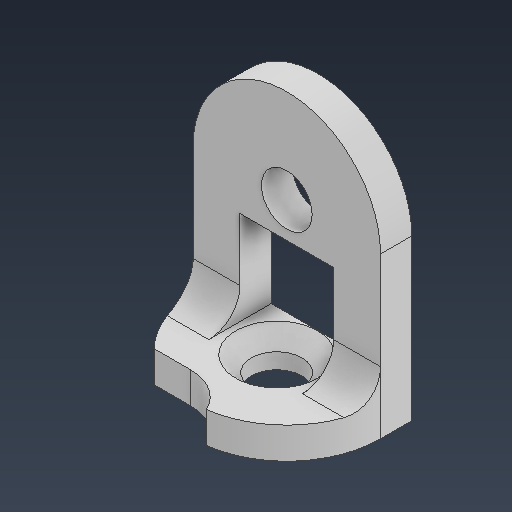
# Autodesk Inventor part: уголок смешной
Saved by Autodesk Inventor 2026 (Build 300175000, 175)
## iProperties
Created: 2026-01-11
Part Number: уголок смешной
Material: Типовые
Document SubType Name: Modeling
Designer: GameHD
Density: 1 g/cm^3
Appearance: По умолчанию
Author: GameHD
Autodesk Inventor part; units mm, degrees
(part 1 of 2)
ref_plane "YZ Plane" through (0, 0, 0) normal (1, 0, 0) x (0, 1, 0)
ref_plane "XZ Plane" through (0, 0, 0) normal (0, 1, 0) x (-1, 0, 0)
ref_plane "XY Plane" through (0, 0, 0) normal (0, 0, 1) x (1, 0, 0)
sketch "Эскиз1" plane through (0, 0, 0) normal (0, 0, 1) x (1, 0, 0)
  circle A0 centre (0, 0) radius 1.625
  line L0 (0, 0) -> (0, -10.25)
  line L1 (-6, 6) -> (6, 6)
  line L2 (6, 6) -> (6, -10.25)
  line L3 (6, -10.25) -> (-6, -10.25)
  line L4 (-6, -10.25) -> (-6, 6)
  line L5 (0, -10.25) -> (-3, -10.25)
  line L6 (-3, -10.25) -> (-3, -4.25)
  line L7 (-3, -4.25) -> (0, -4.25)
  line L8 (0, -4.25) -> (0, -10.25)
  line L9 (3, -10.25) -> (3, -4.25)
  line L10 (3, -4.25) -> (0, -4.25)
  dimension "d0" = 3.25
  dimension "d1" = 10.25
  dimension "d2" = 6
  dimension "d3" = 6
  dimension "d4" = 6
  dimension "d5" = 10.25
  dimension "d6" = 3
  dimension "d7" = 6
  constraints: 22 end point, 4 parallel, 2 horizontal, 2 perpendicular, 2 symmetric about line, 1 centre point, 1 coincident, 1 vertical
  measures "d0" diameter of A0
  measures "d1" distance of L0.start L0.end
  measures "d2" distance from line of L2 L0.start
  measures "d3" distance from line of L4 L0.start
  measures "d4" distance from line of L0.start L1
  measures "d5" distance from line of L0.start L3
  measures "d6" distance of L6.end L7.end
  measures "d7" distance of L5.end L6.end
extrude "Выдавливание1" add sketch "Эскиз1" along normal blind 2 contours L7 L6 L3 L4 L1 L2 L9 L10
sketch "Эскиз2" plane through (0, 0, 2) normal (0, 0, 1) x (1, 0, 0)
  line L0 (3, -4.25) -> (3, -10.25) projected
  line L1 (3, -10.25) -> (6, -10.25) projected
  line L2 (6, -10.25) -> (6, 6) projected
  line L3 (6, 6) -> (-6, 6) projected
  line L4 (-6, 6) -> (-6, -10.25) projected
  line L5 (-6, -10.25) -> (-3, -10.25) projected
  line L6 (-3, -10.25) -> (-3, -4.25) projected
  line L7 (-3, -4.25) -> (3, -4.25) projected
  circle A0 centre (0, 0) radius 1.625 projected
  line L8 (-6, -10.25) -> (6, -10.25)
  line L9 (6, -10.25) -> (6, -8.25)
  line L10 (6, -8.25) -> (-6, -8.25)
  line L11 (-6, -8.25) -> (-6, -10.25)
  dimension "d10" = 12
  dimension "d11" = 2
  constraints: 8 end point, 2 parallel, 1 horizontal, 1 perpendicular
  measures "d10" distance of L10.end L9.end
  measures "d11" distance of L9.end L8.end
extrude "Выдавливание2" add sketch "Эскиз2" along normal blind 6 and the other way blind 2 contours L10 L2 L1 L0 | L0 L8 L6 L10 | L6 L5 L4 L10
sketch "Эскиз3" plane through (-6, -8.25, 2) normal (0, 1, 0) x (1, 0, 0)
  line L0 (0, 0) -> (3, 0) projected
  line L1 (0, -6) -> (0, 0) projected
  line L2 (12, -6) -> (0, -6) projected
  line L3 (12, 0) -> (12, -6) projected
  line L4 (9, 0) -> (12, 0) projected
  line L5 (9, 2) -> (9, 0) projected
  line L6 (3, 2) -> (9, 2) projected
  line L7 (3, 0) -> (3, 2) projected
  circle A0 centre (6, -0.65) radius 1.625
  line L8 (12, 2) -> (0, 2) projected
  point P0 (6, 2)
  point P1 (6, 2)
  dimension "d16" = 3.25
  dimension "d17" = 2.65
  dimension "d20" = 0
  constraints: 1 centre point, 1 midpoint
  measures "d16" diameter of A0
  measures "d17" distance from line of L6 A0.centre
  measures "d20" horizontal distance of point (6, 2) A0.centre
extrude "Выдавливание3" cut sketch "Эскиз3" against normal blind 3.25 contours A0
chamfer "Фаска1" distance 1 angle 45 1 edges at (-1.625, -8.25, 2.65)
fillet "Сопряжение1" radius 6 2 edges at (-6, -9.25, 8) (6, -9.25, 8)
sketch "Эскиз4" plane through (-3, -8.25, 0) normal (0, 1, 0) x (1, 0, 0)
  arc A0 (-244.3999, -16) -> (-248.3999, -20) centre (-244.3999, -20) ccw construction
  line L0 (-244.3999, -16) -> (-177.3999, -16) construction
  arc A1 (-173.3999, -20) -> (-177.3999, -16) centre (-177.3999, -20) ccw construction
  line L1 (-173.3999, -20) -> (-173.3999, -62) construction
  arc A2 (-177.3999, -66) -> (-173.3999, -62) centre (-177.3999, -62) ccw construction
  line L2 (-177.3999, -66) -> (-244.3999, -66) construction
  arc A3 (-248.3999, -62) -> (-244.3999, -66) centre (-244.3999, -62) ccw construction
  line L3 (-248.3999, -62) -> (-248.3999, -20) construction
  line L4 (-244.3999, -336.5) -> (-177.3999, -336.5) construction
  arc A4 (-173.3999, -340.5) -> (-177.3999, -336.5) centre (-177.3999, -340.5) ccw construction
  line L5 (-173.3999, -340.5) -> (-173.3999, -382.5) construction
  arc A5 (-177.3999, -386.5) -> (-173.3999, -382.5) centre (-177.3999, -382.5) ccw construction
  line L6 (-177.3999, -386.5) -> (-244.3999, -386.5) construction
  arc A6 (-248.3999, -382.5) -> (-244.3999, -386.5) centre (-244.3999, -382.5) ccw construction
  line L7 (-248.3999, -382.5) -> (-248.3999, -340.5) construction
  arc A7 (-244.3999, -336.5) -> (-248.3999, -340.5) centre (-244.3999, -340.5) ccw construction
  arc A8 (-136.2796, -72.3282) -> (-139.52, -72.3282) centre (-137.8998, -72.2032) ccw construction
  arc A9 (-139.52, -72.3282) -> (-136.2796, -72.3282) centre (-137.8998, -72.4532) ccw construction
  arc A10 (-365.52, -89.5782) -> (-362.2796, -89.5782) centre (-363.8998, -89.7032) ccw construction
  arc A11 (-362.2796, -89.5782) -> (-365.52, -89.5782) centre (-363.8998, -89.4532) ccw construction
  arc A12 (-225.52, -330.1718) -> (-222.2796, -330.1718) centre (-223.8998, -330.2968) ccw construction
  arc A13 (-222.2796, -330.1718) -> (-225.52, -330.1718) centre (-223.8998, -330.0468) ccw construction
  arc A14 (0.4798, -330.1718) -> (3.7202, -330.1718) centre (2.1, -330.2968) ccw construction
  arc A15 (3.7202, -330.1718) -> (0.4798, -330.1718) centre (2.1, -330.0468) ccw construction
  arc A16 (-136.2796, -312.9218) -> (-139.52, -312.9218) centre (-137.8998, -312.7968) ccw construction
  arc A17 (-139.52, -312.9218) -> (-136.2796, -312.9218) centre (-137.8998, -313.0468) ccw construction
  arc A18 (-362.2796, -312.9218) -> (-365.52, -312.9218) centre (-363.8998, -312.7968) ccw construction
  arc A19 (-365.52, -312.9218) -> (-362.2796, -312.9218) centre (-363.8998, -313.0468) ccw construction
  arc A20 (-225.52, -89.5782) -> (-222.2796, -89.5782) centre (-223.8998, -89.7032) ccw construction
  arc A21 (-222.2796, -89.5782) -> (-225.52, -89.5782) centre (-223.8998, -89.4532) ccw construction
  arc A22 (0.4798, -89.5782) -> (3.7202, -89.5782) centre (2.1, -89.7032) ccw construction
  arc A23 (3.7202, -89.5782) -> (0.4798, -89.5782) centre (2.1, -89.4532) ccw construction
  arc A24 (-139.52, -89.5782) -> (-136.2796, -89.5782) centre (-137.8998, -89.7032) ccw construction
  arc A25 (-136.2796, -89.5782) -> (-139.52, -89.5782) centre (-137.8998, -89.4532) ccw construction
  arc A26 (-362.2796, -72.3282) -> (-365.52, -72.3282) centre (-363.8998, -72.2032) ccw construction
  arc A27 (-365.52, -72.3282) -> (-362.2796, -72.3282) centre (-363.8998, -72.4532) ccw construction
  arc A28 (-222.2796, -312.9218) -> (-225.52, -312.9218) centre (-223.8998, -312.7968) ccw construction
  arc A29 (-225.52, -312.9218) -> (-222.2796, -312.9218) centre (-223.8998, -313.0468) ccw construction
  arc A30 (3.7202, -312.9218) -> (0.4798, -312.9218) centre (2.1, -312.7968) ccw construction
  arc A31 (0.4798, -312.9218) -> (3.7202, -312.9218) centre (2.1, -313.0468) ccw construction
  arc A32 (-139.52, -330.1718) -> (-136.2796, -330.1718) centre (-137.8998, -330.2968) ccw construction
  arc A33 (-136.2796, -330.1718) -> (-139.52, -330.1718) centre (-137.8998, -330.0468) ccw construction
  arc A34 (-365.52, -330.1718) -> (-362.2796, -330.1718) centre (-363.8998, -330.2968) ccw construction
  arc A35 (-362.2796, -330.1718) -> (-365.52, -330.1718) centre (-363.8998, -330.0468) ccw construction
  arc A36 (-222.2796, -72.3282) -> (-225.52, -72.3282) centre (-223.8998, -72.2032) ccw construction
  arc A37 (-225.52, -72.3282) -> (-222.2796, -72.3282) centre (-223.8998, -72.4532) ccw construction
  arc A38 (3.7202, -72.3282) -> (0.4798, -72.3282) centre (2.1, -72.2032) ccw construction
  arc A39 (0.4798, -72.3282) -> (3.7202, -72.3282) centre (2.1, -72.4532) ccw construction
  circle A40 centre (-364.7998, -2.65) radius 1.625 construction
  circle A41 centre (-364.8998, -399.85) radius 1.625 construction
  circle A42 centre (3.0002, -2.65) radius 1.625 construction
  circle A43 centre (3.0002, -399.85) radius 1.625 construction
  circle A44 centre (-180.9846, -7.75) radius 1.625 construction
  circle A45 centre (-180.9846, -394.75) radius 1.625 construction
  circle A46 centre (-223.8998, -7.75) radius 1.625 construction
  circle A47 centre (-223.8998, -394.75) radius 1.625 construction
  circle A48 centre (-124.9057, -203.075) radius 1.85 construction
  arc A49 (-189.2088, -201.25) -> (-188.6026, -201.25) centre (-188.9057, -203.075) ccw construction
  line L8 (-189.2088, -201.25) -> (-188.6026, -201.25) construction
  circle A50 centre (-124.9057, -261.875) radius 2 construction
  circle A51 centre (-308.8939, -169) radius 2.1 construction
  circle A52 centre (-52.9057, -233.5) radius 2.1 construction
  circle A53 centre (-113.9057, -233.5) radius 2.1 construction
  circle A54 centre (-308.8939, -233.5) radius 2.1 construction
  circle A55 centre (-247.8939, -169) radius 2.1 construction
  circle A56 centre (-52.9057, -169) radius 2.1 construction
  circle A57 centre (-113.9057, -169) radius 2.1 construction
  circle A58 centre (-247.8939, -233.5) radius 2.1 construction
  line L9 (-39.8998, -221.25) -> (-3.8998, -221.25) construction
  arc A59 (-0.8998, -224.25) -> (-3.8998, -221.25) centre (-3.8998, -224.25) ccw construction
  line L10 (-0.8998, -224.25) -> (-0.8998, -290.25) construction
  arc A60 (-3.8998, -293.25) -> (-0.8998, -290.25) centre (-3.8998, -290.25) ccw construction
  line L11 (-3.8998, -293.25) -> (-39.8998, -293.25) construction
  arc A61 (-42.8998, -290.25) -> (-39.8998, -293.25) centre (-39.8998, -290.25) ccw construction
  line L12 (-42.8998, -290.25) -> (-42.8998, -224.25) construction
  arc A62 (-39.8998, -221.25) -> (-42.8998, -224.25) centre (-39.8998, -224.25) ccw construction
  circle A63 centre (-160.9, -67.1372) radius 2.1 construction
  circle A64 centre (-52.2429, -99.25) radius 2.1 construction
  circle A65 centre (-160.9, -335.3628) radius 2.1 construction
  circle A66 centre (-52.2429, -212.2592) radius 2.1 construction
  circle A67 centre (-55.8998, -251) radius 2.1 construction
  circle A68 centre (-55.8998, -283.25) radius 2.1 construction
  arc A69 (-25.0518, -344.25) -> (-23.0518, -346.25) centre (-23.0518, -344.25) ccw construction
  line L13 (-23.0518, -346.25) -> (1.1002, -346.25) construction
  arc A70 (4.1002, -349.25) -> (1.1002, -346.25) centre (1.1002, -349.25) ccw construction
  line L14 (4.1002, -349.25) -> (4.1002, -393.25) construction
  arc A71 (1.1002, -396.25) -> (4.1002, -393.25) centre (1.1002, -393.25) ccw construction
  line L15 (1.1002, -396.25) -> (-155.8998, -396.25) construction
  arc A72 (-158.8998, -393.25) -> (-155.8998, -396.25) centre (-155.8998, -393.25) ccw construction
  line L16 (-158.8998, -393.25) -> (-158.8998, -349.25) construction
  arc A73 (-155.8998, -346.25) -> (-158.8998, -349.25) centre (-155.8998, -349.25) ccw construction
  line L17 (-155.8998, -346.25) -> (-107.0518, -346.25) construction
  arc A74 (-107.0518, -346.25) -> (-105.0518, -344.25) centre (-107.0518, -344.25) ccw construction
  line L18 (-105.0518, -344.25) -> (-105.0518, -332.25) construction
  arc A75 (-103.0518, -330.25) -> (-105.0518, -332.25) centre (-103.0518, -332.25) ccw construction
  line L19 (-103.0518, -330.25) -> (-27.0518, -330.25) construction
  arc A76 (-25.0518, -332.25) -> (-27.0518, -330.25) centre (-27.0518, -332.25) ccw construction
  line L20 (-25.0518, -332.25) -> (-25.0518, -344.25) construction
  arc A77 (-338.7478, -346.25) -> (-336.7478, -344.25) centre (-338.7478, -344.25) ccw construction
  line L21 (-336.7478, -344.25) -> (-336.7478, -332.25) construction
  arc A78 (-334.7478, -330.25) -> (-336.7478, -332.25) centre (-334.7478, -332.25) ccw construction
  line L22 (-334.7478, -330.25) -> (-258.7478, -330.25) construction
  arc A79 (-256.7478, -332.25) -> (-258.7478, -330.25) centre (-258.7478, -332.25) ccw construction
  line L23 (-256.7478, -332.25) -> (-256.7478, -394.25) construction
  arc A80 (-258.7478, -396.25) -> (-256.7478, -394.25) centre (-258.7478, -394.25) ccw construction
  line L24 (-258.7478, -396.25) -> (-362.8998, -396.25) construction
  arc A81 (-365.8998, -393.25) -> (-362.8998, -396.25) centre (-362.8998, -393.25) ccw construction
  line L25 (-365.8998, -393.25) -> (-365.8998, -349.25) construction
  arc A82 (-362.8998, -346.25) -> (-365.8998, -349.25) centre (-362.8998, -349.25) ccw construction
  line L26 (-362.8998, -346.25) -> (-338.7478, -346.25) construction
  arc A83 (-336.7478, -58.25) -> (-338.7478, -56.25) centre (-338.7478, -58.25) ccw construction
  line L27 (-338.7478, -56.25) -> (-362.8998, -56.25) construction
  arc A84 (-365.8998, -53.25) -> (-362.8998, -56.25) centre (-362.8998, -53.25) ccw construction
  line L28 (-365.8998, -53.25) -> (-365.8998, -9.25) construction
  arc A85 (-362.8998, -6.25) -> (-365.8998, -9.25) centre (-362.8998, -9.25) ccw construction
  line L29 (-362.8998, -6.25) -> (-258.7478, -6.25) construction
  arc A86 (-256.7478, -8.25) -> (-258.7478, -6.25) centre (-258.7478, -8.25) ccw construction
  line L30 (-256.7478, -8.25) -> (-256.7478, -70.25) construction
  arc A87 (-258.7478, -72.25) -> (-256.7478, -70.25) centre (-258.7478, -70.25) ccw construction
  line L31 (-258.7478, -72.25) -> (-334.7478, -72.25) construction
  arc A88 (-336.7478, -70.25) -> (-334.7478, -72.25) centre (-334.7478, -70.25) ccw construction
  line L32 (-336.7478, -70.25) -> (-336.7478, -58.25) construction
  arc A89 (-23.0518, -56.25) -> (-25.0518, -58.25) centre (-23.0518, -58.25) ccw construction
  line L33 (-25.0518, -58.25) -> (-25.0518, -70.25) construction
  arc A90 (-27.0518, -72.25) -> (-25.0518, -70.25) centre (-27.0518, -70.25) ccw construction
  line L34 (-27.0518, -72.25) -> (-103.0518, -72.25) construction
  arc A91 (-105.0518, -70.25) -> (-103.0518, -72.25) centre (-103.0518, -70.25) ccw construction
  line L35 (-105.0518, -70.25) -> (-105.0518, -58.25) construction
  arc A92 (-105.0518, -58.25) -> (-107.0518, -56.25) centre (-107.0518, -58.25) ccw construction
  line L36 (-107.0518, -56.25) -> (-155.8998, -56.25) construction
  arc A93 (-158.8998, -53.25) -> (-155.8998, -56.25) centre (-155.8998, -53.25) ccw construction
  line L37 (-158.8998, -53.25) -> (-158.8998, -9.25) construction
  arc A94 (-155.8998, -6.25) -> (-158.8998, -9.25) centre (-155.8998, -9.25) ccw construction
  line L38 (-155.8998, -6.25) -> (1.1002, -6.25) construction
  arc A95 (4.1002, -9.25) -> (1.1002, -6.25) centre (1.1002, -9.25) ccw construction
  line L39 (4.1002, -9.25) -> (4.1002, -53.25) construction
  arc A96 (1.1002, -56.25) -> (4.1002, -53.25) centre (1.1002, -53.25) ccw construction
  line L40 (1.1002, -56.25) -> (-23.0518, -56.25) construction
  line L41 (-167.0538, -195.3437) -> (-132.3026, -179.5551) construction
  arc A97 (-128.7277, -184.1712) -> (-132.3026, -179.5551) centre (-131.0617, -182.2864) ccw construction
  line L42 (-128.7277, -184.1712) -> (-141.4776, -199.9598) construction
  arc A98 (-143.8116, -201.075) -> (-141.4776, -199.9598) centre (-143.8116, -198.075) ccw construction
  line L43 (-143.8116, -201.075) -> (-165.8128, -201.075) construction
  arc A99 (-167.0538, -195.3437) -> (-165.8128, -201.075) centre (-165.8128, -198.075) ccw construction
  line L44 (-155.8716, -230.7092) -> (-156.8392, -229.8202) construction
  arc A100 (-157.1435, -225.7262) -> (-156.8392, -229.8202) centre (-154.8095, -227.611) ccw construction
  line L45 (-157.1435, -225.7262) -> (-141.3675, -206.1902) construction
  arc A101 (-139.0335, -205.075) -> (-141.3675, -206.1902) centre (-139.0335, -208.075) ccw construction
  line L46 (-139.0335, -205.075) -> (-136.3621, -205.075) construction
  arc A102 (-133.6126, -206.875) -> (-136.3621, -205.075) centre (-136.3621, -208.075) ccw construction
  arc A103 (-133.6126, -206.875) -> (-128.7057, -211.7819) centre (-124.9057, -203.075) ccw construction
  arc A104 (-126.9057, -214.5314) -> (-128.7057, -211.7819) centre (-129.9057, -214.5314) ccw construction
  line L47 (-126.9057, -214.5314) -> (-126.9057, -228.5) construction
  arc A105 (-129.9057, -231.5) -> (-126.9057, -228.5) centre (-129.9057, -228.5) ccw construction
  line L48 (-129.9057, -231.5) -> (-153.8419, -231.5) construction
  arc A106 (-155.8716, -230.7092) -> (-153.8419, -231.5) centre (-153.8419, -228.5) ccw construction
  line L49 (-181.876, -212.2495) -> (-166.5929, -226.2908) construction
  arc A107 (-168.6226, -231.5) -> (-166.5929, -226.2908) centre (-168.6226, -228.5) ccw construction
  line L50 (-168.6226, -231.5) -> (-183.9057, -231.5) construction
  arc A108 (-186.9057, -228.5) -> (-183.9057, -231.5) centre (-183.9057, -228.5) ccw construction
  line L51 (-186.9057, -228.5) -> (-186.9057, -214.4586) construction
  arc A109 (-181.876, -212.2495) -> (-186.9057, -214.4586) centre (-183.9057, -214.4586) ccw construction
  line L52 (-65.9033, -278.0576) -> (-103.7626, -266.3304) construction
  arc A110 (-103.342, -260.5013) -> (-103.7626, -266.3304) centre (-102.875, -263.4648) ccw construction
  line L53 (-103.342, -260.5013) -> (-65.4826, -254.5349) construction
  arc A111 (-62.0156, -257.4983) -> (-65.4826, -254.5349) centre (-65.0156, -257.4983) ccw construction
  line L54 (-62.0156, -257.4983) -> (-62.0156, -275.192) construction
  arc A112 (-65.9033, -278.0576) -> (-62.0156, -275.192) centre (-65.0156, -275.192) ccw construction
  line L55 (-264.0269, -167) -> (-296.2344, -167) construction
  arc A113 (-298.2843, -161.8097) -> (-296.2344, -167) centre (-296.2344, -164) ccw construction
  line L56 (-298.2843, -161.8097) -> (-284.6652, -149.0634) construction
  arc A114 (-280.9187, -148.7796) -> (-284.6652, -149.0634) centre (-282.6152, -151.2537) ccw construction
  line L57 (-280.9187, -148.7796) -> (-262.3303, -161.5258) construction
  arc A115 (-264.0269, -167) -> (-262.3303, -161.5258) centre (-264.0269, -164) ccw construction
  line L58 (-228.6675, -225.8338) -> (-198.1708, -210.1041) construction
  arc A116 (-194.902, -210.4435) -> (-198.1708, -210.1041) centre (-196.7956, -212.7703) ccw construction
  arc A117 (-194.902, -210.4435) -> (-192.7057, -211.7819) centre (-188.9057, -203.075) ccw construction
  arc A118 (-190.9057, -214.5314) -> (-192.7057, -211.7819) centre (-193.9057, -214.5314) ccw construction
  line L59 (-190.9057, -214.5314) -> (-190.9057, -228.5) construction
  arc A119 (-193.9057, -231.5) -> (-190.9057, -228.5) centre (-193.9057, -228.5) ccw construction
  line L60 (-193.9057, -231.5) -> (-227.2924, -231.5) construction
  arc A120 (-228.6675, -225.8338) -> (-227.2924, -231.5) centre (-227.2924, -228.5) ccw construction
  line L61 (-162.65, -104.8841) -> (-179.1418, -116.8109) construction
  arc A121 (-182.6579, -116.8109) -> (-179.1418, -116.8109) centre (-180.8998, -114.3799) ccw construction
  line L62 (-182.6579, -116.8109) -> (-206.6593, -99.4532) construction
  line L63 (-206.6593, -99.4532) -> (-164.408, -99.4532) construction
  arc A122 (-162.65, -104.8841) -> (-164.408, -99.4532) centre (-164.408, -102.4532) ccw construction
  line L64 (-256.2113, -160.8716) -> (-276.8346, -146.7299) construction
  arc A123 (-277.188, -142.0654) -> (-276.8346, -146.7299) centre (-275.138, -144.2558) ccw construction
  line L65 (-277.188, -142.0654) -> (-236.1047, -103.6152) construction
  arc A124 (-231.1826, -106.6719) -> (-236.1047, -103.6152) centre (-234.0548, -105.8056) ccw construction
  line L66 (-231.1826, -106.6719) -> (-246.5003, -157.4541) construction
  arc A125 (-249.0176, -159.5667) -> (-246.5003, -157.4541) centre (-249.3725, -156.5878) ccw construction
  arc A126 (-249.0176, -159.5667) -> (-252.9258, -160.942) centre (-247.8939, -169) ccw construction
  arc A127 (-256.2113, -160.8716) -> (-252.9258, -160.942) centre (-254.5148, -158.3974) ccw construction
  arc A128 (-65.5653, -167) -> (-63.5153, -161.8097) centre (-65.5653, -164) ccw construction
  line L67 (-65.5653, -167) -> (-102.8117, -167) construction
  arc A129 (-105.0593, -162.013) -> (-102.8117, -167) centre (-102.8117, -164) ccw construction
  line L68 (-105.0593, -162.013) -> (-88.1952, -142.9371) construction
  arc A130 (-83.8976, -142.7337) -> (-88.1952, -142.9371) centre (-85.9475, -144.9241) ccw construction
  line L69 (-83.8976, -142.7337) -> (-63.5153, -161.8097) construction
  line L70 (-243.0573, -104.6436) -> (-281.5342, -140.6545) construction
  arc A131 (-285.2808, -140.9383) -> (-281.5342, -140.6545) centre (-283.5842, -138.4641) ccw construction
  line L71 (-285.2808, -140.9383) -> (-307.5905, -125.6402) construction
  arc A132 (-308.8939, -123.166) -> (-307.5905, -125.6402) centre (-305.8939, -123.166) ccw construction
  line L72 (-308.8939, -123.166) -> (-308.8939, -102.4532) construction
  arc A133 (-305.8939, -99.4532) -> (-308.8939, -102.4532) centre (-305.8939, -102.4532) ccw construction
  line L73 (-305.8939, -99.4532) -> (-245.1073, -99.4532) construction
  arc A134 (-243.0573, -104.6436) -> (-245.1073, -99.4532) centre (-245.1073, -102.4532) ccw construction
  line L74 (-187.6741, -122.9814) -> (-203.7515, -134.6084) construction
  arc A135 (-208.3766, -133.0605) -> (-203.7515, -134.6084) centre (-205.5095, -132.1774) ccw construction
  line L75 (-208.3766, -133.0605) -> (-217.5313, -103.3362) construction
  arc A136 (-214.6642, -99.4532) -> (-217.5313, -103.3362) centre (-214.6642, -102.4532) ccw construction
  line L76 (-214.6642, -99.4532) -> (-214.4563, -99.4532) construction
  arc A137 (-212.6983, -100.0223) -> (-214.4563, -99.4532) centre (-214.4563, -102.4532) ccw construction
  line L77 (-212.6983, -100.0223) -> (-187.6741, -118.1195) construction
  arc A138 (-187.6741, -122.9814) -> (-187.6741, -118.1195) centre (-189.4322, -120.5504) ccw construction
  line L78 (-200.0044, -206.5491) -> (-238.6289, -226.4709) construction
  arc A139 (-241.8976, -226.1315) -> (-238.6289, -226.4709) centre (-240.0041, -223.8047) ccw construction
  arc A140 (-241.8976, -226.1315) -> (-244.0939, -224.7931) centre (-247.8939, -233.5) ccw construction
  arc A141 (-245.8939, -222.0436) -> (-244.0939, -224.7931) centre (-242.8939, -222.0436) ccw construction
  line L79 (-245.8939, -222.0436) -> (-245.8939, -180.4564) construction
  arc A142 (-244.0939, -177.7069) -> (-245.8939, -180.4564) centre (-242.8939, -180.4564) ccw construction
  arc A143 (-244.0939, -177.7069) -> (-242.2553, -176.6456) centre (-247.8939, -169) ccw construction
  arc A144 (-238.9741, -176.4623) -> (-242.2553, -176.6456) centre (-240.4747, -179.0601) ccw construction
  line L80 (-238.9741, -176.4623) -> (-199.8263, -199.0763) construction
  arc A145 (-198.3458, -202.0103) -> (-199.8263, -199.0763) centre (-201.3269, -201.674) ccw construction
  arc A146 (-198.3458, -202.0103) -> (-198.3858, -203.689) centre (-188.9057, -203.075) ccw construction
  arc A147 (-200.0044, -206.5491) -> (-198.3858, -203.689) centre (-201.3796, -203.8829) ccw construction
  line L81 (-281.5342, -261.8455) -> (-240.9203, -299.8564) construction
  arc A148 (-242.9703, -305.0468) -> (-240.9203, -299.8564) centre (-242.9703, -302.0468) ccw construction
  line L82 (-242.9703, -305.0468) -> (-305.8939, -305.0468) construction
  arc A149 (-308.8939, -302.0468) -> (-305.8939, -305.0468) centre (-305.8939, -302.0468) ccw construction
  line L83 (-308.8939, -302.0468) -> (-308.8939, -279.334) construction
  arc A150 (-307.5905, -276.8598) -> (-308.8939, -279.334) centre (-305.8939, -279.334) ccw construction
  line L84 (-307.5905, -276.8598) -> (-285.2808, -261.5617) construction
  arc A151 (-281.5342, -261.8455) -> (-285.2808, -261.5617) centre (-283.5842, -264.0359) ccw construction
  line L85 (-249.8939, -181.5636) -> (-249.8939, -220.9364) construction
  arc A152 (-255.0736, -222.9977) -> (-249.8939, -220.9364) centre (-252.8939, -220.9364) ccw construction
  line L86 (-255.0736, -222.9977) -> (-273.6917, -203.3114) construction
  arc A153 (-273.6917, -199.1886) -> (-273.6917, -203.3114) centre (-271.512, -201.25) ccw construction
  line L87 (-273.6917, -199.1886) -> (-255.0736, -179.5023) construction
  arc A154 (-249.8939, -181.5636) -> (-255.0736, -179.5023) centre (-252.8939, -181.5636) ccw construction
  line L88 (-64.5486, -250.3383) -> (-80.3123, -252.8226) construction
  arc A155 (-81.8793, -247.0681) -> (-80.3123, -252.8226) centre (-80.7793, -249.8592) ccw construction
  line L89 (-81.8793, -247.0681) -> (-66.1156, -240.8557) construction
  arc A156 (-62.0156, -243.6467) -> (-66.1156, -240.8557) centre (-65.0156, -243.6467) ccw construction
  line L90 (-62.0156, -243.6467) -> (-62.0156, -247.3749) construction
  arc A157 (-64.5486, -250.3383) -> (-62.0156, -247.3749) centre (-65.0156, -247.3749) ccw construction
  line L91 (-126.9057, -238.5) -> (-126.9057, -250.4914) construction
  arc A158 (-131.9354, -252.7005) -> (-126.9057, -250.4914) centre (-129.9057, -250.4914) ccw construction
  line L92 (-131.9354, -252.7005) -> (-144.9872, -240.7092) construction
  arc A159 (-142.9575, -235.5) -> (-144.9872, -240.7092) centre (-142.9575, -238.5) ccw construction
  line L93 (-142.9575, -235.5) -> (-129.9057, -235.5) construction
  arc A160 (-126.9057, -238.5) -> (-129.9057, -235.5) centre (-129.9057, -238.5) ccw construction
  line L94 (-178.5975, -175.2286) -> (-185.296, -190.1505) construction
  arc A161 (-190.9, -189.8049) -> (-185.296, -190.1505) centre (-188.0329, -188.9219) ccw construction
  line L95 (-190.9, -189.8049) -> (-195.4958, -174.883) construction
  arc A162 (-192.6287, -171) -> (-195.4958, -174.883) centre (-192.6287, -174) ccw construction
  line L96 (-192.6287, -171) -> (-181.3344, -171) construction
  arc A163 (-178.5975, -175.2286) -> (-181.3344, -171) centre (-181.3344, -174) ccw construction
  line L97 (-87.0478, -216.3052) -> (-75.7345, -201.7118) construction
  arc A164 (-71.6406, -201.094) -> (-75.7345, -201.7118) centre (-73.3635, -203.5499) ccw construction
  line L98 (-71.6406, -201.094) -> (-63.2927, -206.9504) construction
  arc A165 (-62.0156, -209.4063) -> (-63.2927, -206.9504) centre (-65.0156, -209.4063) ccw construction
  line L99 (-62.0156, -209.4063) -> (-62.0156, -211.3707) construction
  arc A166 (-64.0386, -214.2071) -> (-62.0156, -211.3707) centre (-65.0156, -211.3707) ccw construction
  line L100 (-64.0386, -214.2071) -> (-83.6998, -220.9797) construction
  arc A167 (-87.0478, -216.3052) -> (-83.6998, -220.9797) centre (-84.6768, -218.1433) ccw construction
  line L101 (-149.553, -209.9598) -> (-159.8544, -222.7164) construction
  arc A168 (-164.2181, -223.0408) -> (-159.8544, -222.7164) centre (-162.1884, -220.8316) ccw construction
  line L102 (-164.2181, -223.0408) -> (-178.1028, -210.2842) construction
  arc A169 (-176.0732, -205.075) -> (-178.1028, -210.2842) centre (-176.0732, -208.075) ccw construction
  line L103 (-176.0732, -205.075) -> (-151.887, -205.075) construction
  arc A170 (-149.553, -209.9598) -> (-151.887, -205.075) centre (-151.887, -208.075) ccw construction
  line L104 (-79.6231, -190.6077) -> (-99.7954, -176.4559) construction
  arc A171 (-98.0725, -171) -> (-99.7954, -176.4559) centre (-98.0725, -174) ccw construction
  line L105 (-98.0725, -171) -> (-65.0156, -171) construction
  arc A172 (-62.0156, -174) -> (-65.0156, -171) centre (-65.0156, -174) ccw construction
  line L106 (-62.0156, -174) -> (-62.0156, -174.528) construction
  arc A173 (-62.836, -176.5893) -> (-62.0156, -174.528) centre (-65.0156, -174.528) ccw construction
  line L107 (-62.836, -176.5893) -> (-75.7205, -190.2132) construction
  arc A174 (-79.6231, -190.6077) -> (-75.7205, -190.2132) centre (-77.9002, -188.1518) ccw construction
  line L108 (-129.3519, -167) -> (-165.8839, -167) construction
  arc A175 (-168.6208, -162.7714) -> (-165.8839, -167) centre (-165.8839, -164) ccw construction
  line L109 (-168.6208, -162.7714) -> (-159.6674, -142.8267) construction
  arc A176 (-155.1725, -141.6244) -> (-159.6674, -142.8267) centre (-156.9305, -144.0553) ccw construction
  line L110 (-155.1725, -141.6244) -> (-127.5938, -161.5691) construction
  arc A177 (-129.3519, -167) -> (-127.5938, -161.5691) centre (-129.3519, -164) ccw construction
  line L111 (-174.1223, -240.3848) -> (-181.5717, -249.6097) construction
  arc A178 (-186.9057, -247.7249) -> (-181.5717, -249.6097) centre (-183.9057, -247.7249) ccw construction
  line L112 (-186.9057, -247.7249) -> (-186.9057, -238.5) construction
  arc A179 (-183.9057, -235.5) -> (-186.9057, -238.5) centre (-183.9057, -238.5) ccw construction
  line L113 (-183.9057, -235.5) -> (-176.4563, -235.5) construction
  arc A180 (-174.1223, -240.3848) -> (-176.4563, -235.5) centre (-176.4563, -238.5) ccw construction
  line L114 (-95.3944, -295.4734) -> (-120.2601, -304.509) construction
  arc A181 (-124.2847, -301.6894) -> (-120.2601, -304.509) centre (-121.2847, -301.6894) ccw construction
  line L115 (-124.2847, -301.6894) -> (-124.2847, -295.3385) construction
  arc A182 (-121.6067, -292.3558) -> (-124.2847, -295.3385) centre (-121.2847, -295.3385) ccw construction
  line L116 (-121.6067, -292.3558) -> (-96.741, -289.6711) construction
  arc A183 (-95.3944, -295.4734) -> (-96.741, -289.6711) centre (-96.4189, -292.6538) ccw construction
  line L117 (-257.3249, -176.0614) -> (-276.2143, -196.0346) construction
  arc A184 (-280.5736, -196.0346) -> (-276.2143, -196.0346) centre (-278.3939, -193.9732) ccw construction
  line L118 (-280.5736, -196.0346) -> (-299.463, -176.0614) construction
  arc A185 (-297.2834, -171) -> (-299.463, -176.0614) centre (-297.2834, -174) ccw construction
  line L119 (-297.2834, -171) -> (-259.5045, -171) construction
  arc A186 (-257.3249, -176.0614) -> (-259.5045, -171) centre (-259.5045, -174) ccw construction
  line L120 (-67.0656, -153.0084) -> (-81.3715, -139.6194) construction
  arc A187 (-81.5691, -135.442) -> (-81.3715, -139.6194) centre (-79.3215, -137.429) ccw construction
  line L121 (-81.5691, -135.442) -> (-67.2632, -119.2599) construction
  arc A188 (-62.0156, -121.2469) -> (-67.2632, -119.2599) centre (-65.0156, -121.2469) ccw construction
  line L122 (-62.0156, -121.2469) -> (-62.0156, -150.818) construction
  arc A189 (-67.0656, -153.0084) -> (-62.0156, -150.818) centre (-65.0156, -150.818) ccw construction
  line L123 (-124.7239, -158.7082) -> (-154.5063, -137.1698) construction
  arc A190 (-155.4852, -133.5103) -> (-154.5063, -137.1698) centre (-152.7483, -134.7389) ccw construction
  line L124 (-155.4852, -133.5103) -> (-141.5577, -102.4852) construction
  arc A191 (-135.9487, -102.8475) -> (-141.5577, -102.4852) centre (-138.8208, -103.7138) ccw construction
  line L125 (-135.9487, -102.8475) -> (-120.0937, -155.4109) construction
  arc A192 (-124.7239, -158.7082) -> (-120.0937, -155.4109) centre (-122.9659, -156.2773) ccw construction
  line L126 (-62.768, -108.1359) -> (-84.378, -132.5801) construction
  arc A193 (-88.6756, -132.7834) -> (-84.378, -132.5801) centre (-86.6256, -130.593) ccw construction
  line L127 (-88.6756, -132.7834) -> (-118.7424, -104.6436) construction
  arc A194 (-116.6924, -99.4532) -> (-118.7424, -104.6436) centre (-116.6924, -102.4532) ccw construction
  line L128 (-116.6924, -99.4532) -> (-65.0156, -99.4532) construction
  arc A195 (-62.0156, -102.4532) -> (-65.0156, -99.4532) centre (-65.0156, -102.4532) ccw construction
  line L129 (-62.0156, -102.4532) -> (-62.0156, -106.1489) construction
  arc A196 (-62.768, -108.1359) -> (-62.0156, -106.1489) centre (-65.0156, -106.1489) ccw construction
  line L130 (-234.2058, -161.5691) -> (-212.7165, -146.0282) construction
  arc A197 (-208.0914, -147.5761) -> (-212.7165, -146.0282) centre (-210.9585, -148.4591) ccw construction
  line L131 (-208.0914, -147.5761) -> (-203.305, -163.117) construction
  arc A198 (-206.1721, -167) -> (-203.305, -163.117) centre (-206.1721, -164) ccw construction
  line L132 (-206.1721, -167) -> (-232.4478, -167) construction
  arc A199 (-234.2058, -161.5691) -> (-232.4478, -167) centre (-232.4478, -164) ccw construction
  line L133 (-198.5757, -164.883) -> (-205.2681, -143.1534) construction
  arc A200 (-204.159, -139.8395) -> (-205.2681, -143.1534) centre (-202.401, -142.2704) ccw construction
  line L134 (-204.159, -139.8395) -> (-182.6579, -124.29) construction
  arc A201 (-179.1418, -124.29) -> (-182.6579, -124.29) centre (-180.8998, -126.721) ccw construction
  line L135 (-179.1418, -124.29) -> (-163.4475, -135.6401) construction
  arc A202 (-162.4686, -139.2996) -> (-163.4475, -135.6401) centre (-165.2055, -138.071) ccw construction
  line L136 (-162.4686, -139.2996) -> (-174.1084, -165.2286) construction
  arc A203 (-176.8453, -167) -> (-174.1084, -165.2286) centre (-176.8453, -164) ccw construction
  line L137 (-176.8453, -167) -> (-195.7086, -167) construction
  arc A204 (-198.5757, -164.883) -> (-195.7086, -167) centre (-195.7086, -164) ccw construction
  line L138 (-276.2143, -206.4654) -> (-257.3249, -226.4386) construction
  arc A205 (-259.5045, -231.5) -> (-257.3249, -226.4386) centre (-259.5045, -228.5) ccw construction
  line L139 (-259.5045, -231.5) -> (-297.2834, -231.5) construction
  arc A206 (-299.463, -226.4386) -> (-297.2834, -231.5) centre (-297.2834, -228.5) ccw construction
  line L140 (-299.463, -226.4386) -> (-280.5736, -206.4654) construction
  arc A207 (-276.2143, -206.4654) -> (-280.5736, -206.4654) centre (-278.3939, -208.5268) ccw construction
  line L141 (-301.7143, -179.5023) -> (-283.0962, -199.1886) construction
  arc A208 (-283.0962, -203.3114) -> (-283.0962, -199.1886) centre (-285.2758, -201.25) ccw construction
  line L142 (-283.0962, -203.3114) -> (-301.7143, -222.9977) construction
  arc A209 (-306.8939, -220.9364) -> (-301.7143, -222.9977) centre (-303.8939, -220.9364) ccw construction
  line L143 (-306.8939, -220.9364) -> (-306.8939, -181.5636) construction
  arc A210 (-301.7143, -179.5023) -> (-306.8939, -181.5636) centre (-303.8939, -181.5636) ccw construction
  line L144 (-181.6607, -191.8194) -> (-173.1099, -172.7714) construction
  arc A211 (-170.373, -171) -> (-173.1099, -172.7714) centre (-170.373, -174) ccw construction
  line L145 (-170.373, -171) -> (-136.9986, -171) construction
  arc A212 (-135.7576, -176.7313) -> (-136.9986, -171) centre (-136.9986, -174) ccw construction
  line L146 (-135.7576, -176.7313) -> (-177.6829, -195.7794) construction
  arc A213 (-181.6607, -191.8194) -> (-177.6829, -195.7794) centre (-178.9238, -193.048) ccw construction
  line L147 (-112.1678, -248.7083) -> (-102.829, -236.6619) construction
  arc A214 (-100.4581, -235.5) -> (-102.829, -236.6619) centre (-100.4581, -238.5) ccw construction
  line L148 (-100.4581, -235.5) -> (-79.2299, -235.5) construction
  arc A215 (-78.1299, -241.2911) -> (-79.2299, -235.5) centre (-79.2299, -238.5) ccw construction
  line L149 (-78.1299, -241.2911) -> (-108.6969, -253.3374) construction
  arc A216 (-112.1678, -248.7083) -> (-108.6969, -253.3374) centre (-109.7968, -250.5464) ccw construction
  line L150 (-105.6757, -177.2168) -> (-83.1221, -193.0392) construction
  arc A217 (-82.6654, -197.5565) -> (-83.1221, -193.0392) centre (-84.845, -195.4951) ccw construction
  line L151 (-82.6654, -197.5565) -> (-106.7261, -222.9977) construction
  arc A218 (-111.9057, -220.9364) -> (-106.7261, -222.9977) centre (-108.9057, -220.9364) ccw construction
  line L152 (-111.9057, -220.9364) -> (-111.9057, -180.4564) construction
  arc A219 (-110.1057, -177.7069) -> (-111.9057, -180.4564) centre (-108.9057, -180.4564) ccw construction
  arc A220 (-110.1057, -177.7069) -> (-108.9603, -177.1113) centre (-113.9057, -169) ccw construction
  arc A221 (-105.6757, -177.2168) -> (-108.9603, -177.1113) centre (-107.3986, -179.6727) ccw construction
  line L153 (-276.8346, -255.7701) -> (-274.329, -254.0519) construction
  arc A222 (-271.33, -253.8236) -> (-274.329, -254.0519) centre (-272.6324, -256.5261) ccw construction
  line L154 (-271.33, -253.8236) -> (-232.9823, -272.3047) construction
  arc A223 (-231.2847, -275.0072) -> (-232.9823, -272.3047) centre (-234.2847, -275.0072) ccw construction
  line L155 (-231.2847, -275.0072) -> (-231.2847, -296.4793) construction
  arc A224 (-236.3347, -298.6696) -> (-231.2847, -296.4793) centre (-234.2847, -296.4793) ccw construction
  line L156 (-236.3347, -298.6696) -> (-277.188, -260.4346) construction
  arc A225 (-276.8346, -255.7701) -> (-277.188, -260.4346) centre (-275.138, -258.2442) ccw construction
  line L157 (-130.2847, -280.5) -> (-130.2847, -304.5) construction
  arc A226 (-133.2847, -307.5) -> (-130.2847, -304.5) centre (-133.2847, -304.5) ccw construction
  line L158 (-133.2847, -307.5) -> (-222.2847, -307.5) construction
  arc A227 (-225.2847, -304.5) -> (-222.2847, -307.5) centre (-222.2847, -304.5) ccw construction
  line L159 (-225.2847, -304.5) -> (-225.2847, -280.5) construction
  arc A228 (-222.2847, -277.5) -> (-225.2847, -280.5) centre (-222.2847, -280.5) ccw construction
  line L160 (-222.2847, -277.5) -> (-133.2847, -277.5) construction
  arc A229 (-130.2847, -280.5) -> (-133.2847, -277.5) centre (-133.2847, -280.5) ccw construction
  line L161 (-125.6949, -103.6152) -> (-91.2017, -135.8978) construction
  arc A230 (-91.004, -140.0751) -> (-91.2017, -135.8978) centre (-93.2516, -138.0881) ccw construction
  line L162 (-91.004, -140.0751) -> (-107.8161, -159.0921) construction
  arc A231 (-110.9858, -159.9599) -> (-107.8161, -159.0921) centre (-110.0637, -157.1051) ccw construction
  arc A232 (-110.9858, -159.9599) -> (-112.782, -159.5667) centre (-113.9057, -169) ccw construction
  arc A233 (-115.2994, -157.4541) -> (-112.782, -159.5667) centre (-112.4272, -156.5878) ccw construction
  line L163 (-115.2994, -157.4541) -> (-130.6171, -106.6719) construction
  arc A234 (-125.6949, -103.6152) -> (-130.6171, -106.6719) centre (-127.7449, -105.8056) ccw construction
  arc A235 (-124.0421, -273.0589) -> (-124.2847, -275.0142) centre (-116.2847, -275.0142) ccw construction
  arc A236 (-122.0385, -270.932) -> (-124.0421, -273.0589) centre (-121.1331, -273.7921) ccw construction
  arc A237 (-122.0385, -270.932) -> (-117.7388, -268.1108) centre (-124.9057, -261.875) ccw construction
  arc A238 (-114.9901, -267.1196) -> (-117.7388, -268.1108) centre (-115.4756, -270.0801) ccw construction
  arc A239 (-113.9176, -267.3724) -> (-114.9901, -267.1196) centre (-116.2847, -275.0142) ccw construction
  line L164 (-113.9176, -267.3724) -> (-79.5821, -278.008) construction
  arc A240 (-80.1478, -283.8563) -> (-79.5821, -278.008) centre (-80.4698, -280.8737) ccw construction
  line L165 (-80.1478, -283.8563) -> (-120.9627, -288.263) construction
  arc A241 (-124.2847, -285.2803) -> (-120.9627, -288.263) centre (-121.2847, -285.2803) ccw construction
  line L166 (-124.2847, -285.2803) -> (-124.2847, -275.0142) construction
  line L167 (-85.0153, -225.6636) -> (-65.9927, -219.1109) construction
  arc A242 (-62.0156, -221.9473) -> (-65.9927, -219.1109) centre (-65.0156, -221.9473) ccw construction
  line L168 (-62.0156, -221.9473) -> (-62.0156, -228.5) construction
  arc A243 (-65.0156, -231.5) -> (-62.0156, -228.5) centre (-65.0156, -228.5) ccw construction
  line L169 (-65.0156, -231.5) -> (-84.0383, -231.5) construction
  arc A244 (-85.0153, -225.6636) -> (-84.0383, -231.5) centre (-84.0383, -228.5) ccw construction
  line L170 (-220.9829, -105.7189) -> (-211.1999, -137.4831) construction
  arc A245 (-212.309, -140.7971) -> (-211.1999, -137.4831) centre (-214.067, -138.3662) ccw construction
  line L171 (-212.309, -140.7971) -> (-237.0758, -158.7082) construction
  arc A246 (-241.706, -155.4109) -> (-237.0758, -158.7082) centre (-238.8338, -156.2773) ccw construction
  line L172 (-241.706, -155.4109) -> (-226.7222, -105.7356) construction
  arc A247 (-220.9829, -105.7189) -> (-226.7222, -105.7356) centre (-223.85, -106.602) ccw construction
  arc A248 (-180.8497, -266.91) -> (-180.1988, -265.675) centre (-188.9057, -261.875) ccw construction
  arc A249 (-177.4493, -263.875) -> (-180.1988, -265.675) centre (-177.4493, -266.875) ccw construction
  line L173 (-177.4493, -263.875) -> (-141.8098, -263.875) construction
  arc A250 (-140.1779, -269.3923) -> (-141.8098, -263.875) centre (-141.8098, -266.875) ccw construction
  line L174 (-140.1779, -269.3923) -> (-142.6844, -271.0173) construction
  arc A251 (-144.3164, -271.5) -> (-142.6844, -271.0173) centre (-144.3164, -268.5) ccw construction
  line L175 (-144.3164, -271.5) -> (-178.3057, -271.5) construction
  arc A252 (-180.8497, -266.91) -> (-178.3057, -271.5) centre (-178.3057, -268.5) ccw construction
  arc A253 (-198.2534, -263.5693) -> (-196.9617, -266.91) centre (-188.9057, -261.875) ccw construction
  arc A254 (-199.5057, -271.5) -> (-196.9617, -266.91) centre (-199.5057, -268.5) ccw construction
  line L176 (-199.5057, -271.5) -> (-224.7534, -271.5) construction
  arc A255 (-226.0559, -271.2025) -> (-224.7534, -271.5) centre (-224.7534, -268.5) ccw construction
  line L177 (-226.0559, -271.2025) -> (-264.428, -252.7096) construction
  arc A256 (-264.8221, -247.5329) -> (-264.428, -252.7096) centre (-263.1255, -250.0071) ccw construction
  line L178 (-264.8221, -247.5329) -> (-264.2302, -247.1271) construction
  arc A257 (-261.8433, -246.6818) -> (-264.2302, -247.1271) centre (-262.5337, -249.6013) ccw construction
  line L179 (-261.8433, -246.6818) -> (-200.5149, -261.1848) construction
  arc A258 (-198.2534, -263.5693) -> (-200.5149, -261.1848) centre (-201.2053, -264.1043) ccw construction
  line L180 (-180.152, -254.2184) -> (-165.9368, -236.6152) construction
  arc A259 (-163.6028, -235.5) -> (-165.9368, -236.6152) centre (-163.6028, -238.5) ccw construction
  line L181 (-163.6028, -235.5) -> (-156.5693, -235.5) construction
  line L182 (-156.5693, -235.5) -> (-135.7086, -254.6658) construction
  arc A260 (-137.7382, -259.875) -> (-135.7086, -254.6658) centre (-137.7382, -256.875) ccw construction
  line L183 (-137.7382, -259.875) -> (-177.4493, -259.875) construction
  arc A261 (-180.1988, -258.075) -> (-177.4493, -259.875) centre (-177.4493, -256.875) ccw construction
  arc A262 (-180.1988, -258.075) -> (-180.4791, -257.4884) centre (-188.9057, -261.875) ccw construction
  arc A263 (-180.152, -254.2184) -> (-180.4791, -257.4884) centre (-177.818, -256.1032) ccw construction
  line L184 (-198.3628, -255.1065) -> (-227.2655, -241.2035) construction
  arc A264 (-225.9651, -235.5) -> (-227.2655, -241.2035) centre (-225.9651, -238.5) ccw construction
  line L185 (-225.9651, -235.5) -> (-193.9057, -235.5) construction
  arc A265 (-190.9057, -238.5) -> (-193.9057, -235.5) centre (-193.9057, -238.5) ccw construction
  line L186 (-190.9057, -238.5) -> (-190.9057, -250.4186) construction
  arc A266 (-192.7057, -253.1681) -> (-190.9057, -250.4186) centre (-193.9057, -250.4186) ccw construction
  arc A267 (-192.7057, -253.1681) -> (-195.1048, -254.6763) centre (-188.9057, -261.875) ccw construction
  arc A268 (-198.3628, -255.1065) -> (-195.1048, -254.6763) centre (-197.0624, -252.403) ccw construction
  line L187 (-229.2423, -171) -> (-203.0922, -171) construction
  arc A269 (-200.2251, -173.117) -> (-203.0922, -171) centre (-203.0922, -174) ccw construction
  line L188 (-200.2251, -173.117) -> (-194.5659, -191.4919) construction
  arc A270 (-198.9336, -194.9726) -> (-194.5659, -191.4919) centre (-197.433, -192.3749) ccw construction
  line L189 (-198.9336, -194.9726) -> (-230.7429, -176.5977) construction
  arc A271 (-229.2423, -171) -> (-230.7429, -176.5977) centre (-229.2423, -174) ccw construction
  circle A272 centre (-188.9057, -261.875) radius 2 construction
  line L190 (-308.8939, -156.8653) -> (-308.8939, -135.2912) construction
  arc A273 (-304.1974, -132.817) -> (-308.8939, -135.2912) centre (-305.8939, -135.2912) ccw construction
  line L191 (-304.1974, -132.817) -> (-289.3648, -142.9879) construction
  arc A274 (-289.0114, -147.6525) -> (-289.3648, -142.9879) centre (-291.0614, -145.4621) ccw construction
  line L192 (-289.0114, -147.6525) -> (-301.896, -159.7113) construction
  arc A275 (-305.1335, -160.2759) -> (-301.896, -159.7113) centre (-303.946, -157.521) ccw construction
  arc A276 (-305.1335, -160.2759) -> (-306.6139, -159.7777) centre (-308.8939, -169) ccw construction
  arc A277 (-308.8939, -156.8653) -> (-306.6139, -159.7777) centre (-305.8939, -156.8653) ccw construction
  line L193 (-308.8939, -267.2088) -> (-308.8939, -245.6347) construction
  arc A278 (-306.6139, -242.7223) -> (-308.8939, -245.6347) centre (-305.8939, -245.6347) ccw construction
  arc A279 (-306.6139, -242.7223) -> (-305.1335, -242.2241) centre (-308.8939, -233.5) ccw construction
  arc A280 (-301.896, -242.7887) -> (-305.1335, -242.2241) centre (-303.946, -244.979) ccw construction
  line L194 (-301.896, -242.7887) -> (-289.0114, -254.8475) construction
  arc A281 (-289.3648, -259.5121) -> (-289.0114, -254.8475) centre (-291.0614, -257.0379) ccw construction
  line L195 (-289.3648, -259.5121) -> (-304.1974, -269.683) construction
  arc A282 (-308.8939, -267.2088) -> (-304.1974, -269.683) centre (-305.8939, -267.2088) ccw construction
  line L196 (-147.3798, -105.6875) -> (-158.2864, -129.9831) construction
  arc A283 (-162.7813, -131.1854) -> (-158.2864, -129.9831) centre (-161.0232, -128.7545) ccw construction
  line L197 (-162.7813, -131.1854) -> (-174.1255, -122.9814) construction
  arc A284 (-174.1255, -118.1195) -> (-174.1255, -122.9814) centre (-172.3675, -120.5504) ccw construction
  line L198 (-174.1255, -118.1195) -> (-151.8747, -102.0279) construction
  arc A285 (-147.3798, -105.6875) -> (-151.8747, -102.0279) centre (-150.1167, -104.4588) ccw construction
  circle A286 centre (4.1002, -233.5) radius 1.5 construction
  circle A287 centre (4.1002, -275.192) radius 1.5 construction
  line L199 (-44.2909, -212.171) -> (-45.7001, -211.8215) construction
  arc A288 (-47.7022, -210.1658) -> (-45.7001, -211.8215) centre (-44.9778, -208.9097) ccw construction
  arc A289 (-47.7022, -210.1658) -> (-47.8057, -209.9545) centre (-52.2429, -212.2592) ccw construction
  arc A290 (-47.8868, -207.3577) -> (-47.8057, -209.9545) centre (-45.1434, -208.5717) ccw construction
  line L200 (-47.8868, -207.3577) -> (-41.0124, -191.8227) construction
  arc A291 (-36.0247, -191.046) -> (-41.0124, -191.8227) centre (-38.269, -193.0367) ccw construction
  line L201 (-36.0247, -191.046) -> (-21.6355, -207.2685) construction
  arc A292 (-23.8799, -212.2592) -> (-21.6355, -207.2685) centre (-23.8799, -209.2592) ccw construction
  line L202 (-23.8799, -212.2592) -> (-43.5687, -212.2592) construction
  arc A293 (-44.2909, -212.171) -> (-43.5687, -212.2592) centre (-43.5687, -209.2592) ccw construction
  line L203 (-32.0299, -142.3268) -> (-26.357, -134.1229) construction
  arc A294 (-21.1461, -137.0431) -> (-26.357, -134.1229) centre (-23.8895, -135.8291) ccw construction
  line L204 (-21.1461, -137.0431) -> (-25.8664, -147.7102) construction
  arc A295 (-31.4078, -147.5784) -> (-25.8664, -147.7102) centre (-28.6098, -146.4962) ccw construction
  line L205 (-31.4078, -147.5784) -> (-32.3604, -145.1152) construction
  arc A296 (-32.0299, -142.3268) -> (-32.3604, -145.1152) centre (-29.5624, -144.033) ccw construction
  line L206 (-44.6931, -124.316) -> (-38.0013, -141.619) construction
  arc A297 (-38.3318, -144.4074) -> (-38.0013, -141.619) centre (-40.7993, -142.7011) ccw construction
  line L207 (-38.3318, -144.4074) -> (-45.2836, -154.4608) construction
  arc A298 (-50.751, -152.726) -> (-45.2836, -154.4608) centre (-47.7511, -152.7545) ccw construction
  line L208 (-50.751, -152.726) -> (-50.491, -125.3696) construction
  arc A299 (-44.6931, -124.316) -> (-50.491, -125.3696) centre (-47.4911, -125.3981) ccw construction
  arc A300 (-47.9779, -169.8463) -> (-48.1155, -167.567) centre (-52.9057, -169) ccw construction
  arc A301 (-47.7088, -165.001) -> (-48.1155, -167.567) centre (-45.2413, -166.7072) ccw construction
  line L209 (-47.7088, -165.001) -> (-38.906, -152.2706) construction
  arc A302 (-33.6404, -152.8948) -> (-38.906, -152.2706) centre (-36.4385, -153.9769) ccw construction
  line L210 (-33.6404, -152.8948) -> (-31.5331, -158.3436) construction
  arc A303 (-31.5878, -160.6397) -> (-31.5331, -158.3436) centre (-34.3312, -159.4257) ccw construction
  line L211 (-31.5878, -160.6397) -> (-38.3722, -175.9713) construction
  arc A304 (-43.3599, -176.7481) -> (-38.3722, -175.9713) centre (-41.1156, -174.7574) ccw construction
  line L212 (-43.3599, -176.7481) -> (-47.2655, -172.3448) construction
  arc A305 (-47.9779, -169.8463) -> (-47.2655, -172.3448) centre (-45.0212, -170.3541) ccw construction
  line L213 (-45.4554, -180.4136) -> (-43.3203, -182.8208) construction
  arc A306 (-42.8212, -186.0255) -> (-43.3203, -182.8208) centre (-45.5646, -184.8115) ccw construction
  line L214 (-42.8212, -186.0255) -> (-44.8492, -190.6084) construction
  arc A307 (-50.5923, -189.4404) -> (-44.8492, -190.6084) centre (-47.5926, -189.3944) ccw construction
  line L215 (-50.5923, -189.4404) -> (-50.6994, -182.4503) construction
  arc A308 (-45.4554, -180.4136) -> (-50.6994, -182.4503) centre (-47.6998, -182.4043) ccw construction
  line L216 (-1.0791, -115.8997) -> (-1.0791, -199.649) construction
  arc A309 (-1.5533, -201.2676) -> (-1.0791, -199.649) centre (-4.0791, -199.649) ccw construction
  arc A310 (-9.2686, -202.8487) -> (-1.5533, -201.2676) centre (-6.1806, -198.3022) ccw construction
  arc A311 (-10.6329, -201.2956) -> (-9.2686, -202.8487) centre (-7.8349, -200.2135) ccw construction
  line L217 (-10.6329, -201.2956) -> (-26.3078, -160.7653) construction
  arc A312 (-26.2532, -158.4692) -> (-26.3078, -160.7653) centre (-23.5098, -159.6832) ccw construction
  line L218 (-26.2532, -158.4692) -> (-6.8196, -114.5524) construction